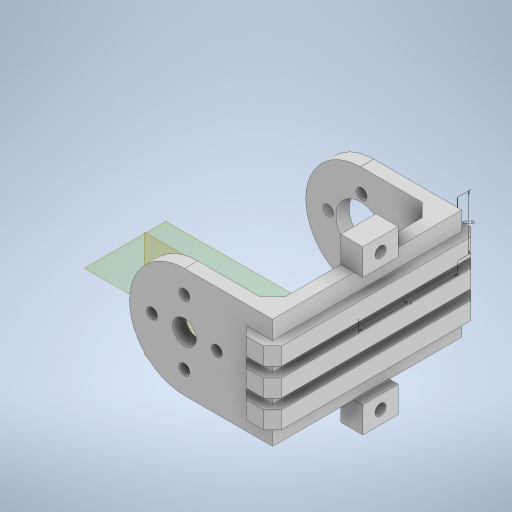
# Autodesk Inventor part: UnionCuerpo
Saved by Autodesk Inventor 2024 (Build 280153000, 153)
## iProperties
Created: 2024-03-17
Part Number: UnionCuerpo
Material: Genérico
Document SubType Name: Modeling
Designer: na_re
Density: 1 g/cm^3
Appearance: Valor por defecto
Author: na_re
Autodesk Inventor part; units mm, degrees
ref_plane "YZ Plane" through (0, 0, 0) normal (1, 0, 0) x (0, 1, 0)
ref_plane "XZ Plane" through (0, 0, 0) normal (0, 1, 0) x (-1, 0, 0)
ref_plane "XY Plane" through (0, 0, 0) normal (0, 0, 1) x (1, 0, 0)
ref_plane "Plano de trabajo1" through (0, 0, 0) normal (0, 0, 1) x (1, 0, 0)
sketch "Boceto1" plane through (0, 0, 0) normal (0, 0, 1) x (1, 0, 0)
  circle A0 centre (18.3423, 0) radius 1.2028 projected
  circle A1 centre (3.6423, 0) radius 1.2028 projected
  circle A2 centre (10.9923, -7.35) radius 1.2028 projected
  circle A3 centre (10.9923, 7.35) radius 1.2028 projected
  circle A4 centre (10.9923, 0) radius 10.9823 projected
  circle A5 centre (10.9923, 0) radius 2.7 projected
  circle A6 centre (10.9923, 0) radius 12.5
  line L0 (10.9923, 0) -> (22.9923, 0)
  line L1 (10.9923, 0) -> (10.9923, 12.5)
  line L2 (10.9923, 12.5) -> (22.9923, 12.5)
  line L3 (10.9923, 0) -> (10.9923, -12.5)
  line L4 (10.9923, -12.5) -> (22.9923, -12.5)
  line L5 (22.9923, -12.5) -> (22.9923, 12.5)
  point P0 (0, 0)
  dimension "d0" = 25
  dimension "d1" = 12
  dimension "d2" = 12
  constraints: 12 end point, 2 horizontal, 2 perpendicular, 2 point on circle, 2 vertical, 1 centre point, 1 coincident, 1 tangent
  measures "d0" diameter of A6
  measures "d1" distance of L0.start L0.end
  measures "d2" distance of L1.end L2.end
extrude "Extrusión1" add sketch "Boceto1" along normal blind 3 contours L0 A4 L3 A2 A5 A0 | A0 L0 A5 L1 A3 A4 | L0 L5 A6 L3 A4 | A4 L1 A6 L5 L0 | L1 A3 A5 L3 A2 A4 | A4 L3 A6 L1 | L2 L5 A6 | A6 L5 L4
sketch "Boceto2" plane through (22.9923, -12.5, 0) normal (1, 0, 0) x (0, 0, -1)
  line L0 (0, 0) -> (0, 25) projected
  line L1 (0, 25) -> (-3, 25) projected
  line L2 (-3, 0) -> (-3, 25) projected
  line L3 (0, 0) -> (-3, 0) projected
  point P0 (0, 12.5)
extrude "Extrusión2" add sketch "Boceto2" along normal blind 8
sketch "Boceto3" plane through (0, 0, 0) normal (0, 0, -1) x (-1, 0, 0)
  line L0 (-10.9923, -12.5) -> (-30.9923, -12.5) projected
  arc A0 (-10.9923, -12.5) -> (-10.9923, 12.5) centre (-10.9923, 0) ccw projected
  line L1 (-10.9923, 12.5) -> (-30.9923, 12.5) projected
  line L2 (-30.9923, -12.5) -> (-30.9923, 12.5) projected
  circle A1 centre (-10.9923, 0) radius 2.7 projected
  circle A2 centre (-10.9923, 7.35) radius 1.2028 projected
  circle A3 centre (-18.3423, 0) radius 1.2028 projected
  circle A4 centre (-3.6423, 0) radius 1.2028 projected
  circle A5 centre (-10.9923, -7.35) radius 1.2028 projected
  line L3 (-30.9923, 12.5) -> (-27.9923, 12.5)
  line L4 (-27.9923, 12.5) -> (-27.9923, -12.5)
  line L5 (-27.9923, -12.5) -> (-30.9923, -12.5)
  line L6 (-30.9923, -12.5) -> (-30.9923, 12.5)
  point P0 (0, 0)
  dimension "d7" = 3
  constraints: 8 end point, 2 parallel, 1 horizontal, 1 perpendicular, 1 point on line
  measures "d7" distance of L4.end L5.end
extrude "Extrusión3" add sketch "Boceto3" along normal blind 42 contours L0 L2 L1 L4
sketch "Boceto4" plane through (27.9923, -12.5, 0) normal (-1, 0, 0) x (0, 0, 1)
  line L0 (-42, 0) -> (-42, 25) projected
  line L1 (0, 25) -> (0, 0) projected
  line L2 (0, 25) -> (-42, 25) projected
  line L3 (-42, 0) -> (-42, 25) projected
  line L4 (0, 0) -> (-42, 0) projected
  line L5 (-42, 0) -> (-40, 0)
  line L6 (-40, 0) -> (-40, 25)
  line L7 (-40, 25) -> (-42, 25)
  line L8 (-42, 25) -> (-42, 0)
  point P0 (0, 12.5)
  dimension "d10" = 2
  constraints: 8 end point, 2 parallel, 1 horizontal, 1 perpendicular, 1 point on line
  measures "d10" distance of L7.end L6.end
extrude "Extrusión4" add sketch "Boceto4" along normal blind 30 contours L0 L2 L6 L4
sketch "Boceto5" plane through (0, 0, -42) normal (0, 0, -1) x (-1, 0, 0)
  line L0 (24.4501, 12.6367) -> (24.5578, -12.3277) projected
  line L1 (-11.0672, 12.4835) -> (24.4501, 12.6367) projected
  arc A0 (-11.0672, 12.4835) -> (-10.9596, -12.4809) centre (-11.0134, 0.0013) ccw projected
  line L2 (-10.9596, -12.4809) -> (24.5578, -12.3277) projected
  circle A1 centre (-3.6676, 0.2495) radius 1.2028 projected
  circle A2 centre (-11.0134, 0.0013) radius 2.7 projected
  circle A3 centre (-10.7652, -7.3445) radius 1.2028 projected
  circle A4 centre (-11.2616, 7.3471) radius 1.2028 projected
  circle A5 centre (-18.3592, -0.2469) radius 1.2028 projected
  line L3 (-30.9923, 12.5) -> (2.0077, 12.5) projected
  line L4 (-11.0672, 12.4835) -> (2.0077, 12.5)
  line L5 (2.0391, -12.4248) -> (2.0077, 12.5)
  line L6 (-10.9596, -12.4809) -> (2.0391, -12.4248)
  line L7 (-11.0672, 12.4835) -> (2.0077, 12.5)
  circle A6 centre (-11.0134, 0.0013) radius 12.4823
  line L8 (-10.7652, -7.3445) -> (-10.7652, -14.8497)
  line L9 (-10.7652, -14.8497) -> (6.2045, -14.8497)
  line L10 (6.2045, -14.8497) -> (6.2045, 15.7882)
  line L11 (6.2045, 15.7882) -> (-10.7652, 15.7882)
  line L12 (-10.7652, 15.7882) -> (-11.2616, 7.3471)
  point P0 (0, 0)
  point P1 (-7.2489, 12.5)
  point P2 (-10.991, 12.4836)
  point P3 (-10.9817, -12.481)
  point P4 (-10.9586, 12.5)
  point P5 (6.2045, 12.558)
  point P6 (6.2045, -12.4069)
  point P7 (-10.7652, -12.48)
  point P8 (-10.9595, 12.484)
  point P9 (-10.9595, 12.4837)
  point P10 (-10.9596, 12.4835)
  point P11 (-10.991, 12.4836)
  point P12 (-10.7652, -12.4785)
  point P13 (-11.0672, 12.4835)
  constraints: 18 end point, 4 perpendicular, 2 point on line, 1 coincident, 1 collinear, 1 vertical, 3 other
extrude "Extrusión5" cut sketch "Boceto5" against normal blind 25 contours L10 L2 L5 L3 L1 | L1 L3 L12 L11 L10 | L10 L9 L8 L2 | L3 L4 L1 | L1 L12 L3 | L2 A6 L4 L5 | A1 | A2 | A3 | A4 | A5
sketch "Boceto8" plane through (10.9923, -12.5, 0) normal (0, -1, 0) x (1, 0, 0)
  line L0 (-0.2271, -40) -> (-0.2271, -42) projected
  line L1 (20, -42) -> (-0.2271, -42) projected
  line L2 (20, 3) -> (20, -42) projected
  line L3 (0, 3) -> (20, 3) projected
  line L4 (0, 0) -> (0, 3) projected
  line L5 (0, 0) -> (17, 0) projected
  line L6 (17, 0) -> (17, -40) projected
  line L7 (17, -40) -> (-0.2271, -40) projected
  line L8 (20, -42) -> (20, -19.5)
  line L9 (20, 3) -> (20, -42) projected
  line L10 (20, -19.5) -> (20, -23.5)
  line L11 (20, -23.5) -> (20, -15.5)
  line L12 (20, -15.5) -> (17, -15.5)
  line L13 (20, -23.5) -> (17, -23.5)
  point P0 (-10.9923, 0)
  dimension "d29" = 22.5
  dimension "d30" = 4
  dimension "d31" = 8
  constraints: 10 end point, 4 point on line, 2 perpendicular, 1 midpoint
  measures "d29" distance of L1.start L8.end
  measures "d30" distance of L8.end L10.end
  measures "d31" distance of L10.end L11.end
extrude "Extrusión8" add sketch "Boceto8" along normal blind 6 contours L6 L12 L2 L13
ref_plane "Plano de trabajo2" through (-0.8313, -11.6464, -27.56) normal (0.0047593, -0.9999887, 0) x (0.9999887, 0.0047593, 0)
sketch "Boceto9" plane through (30.9923, -12.5, 0) normal (1, 0, 0) x (0, 0, -1)
  line L0 (-3, 25) -> (42, 25) projected
  line L1 (-3, 25) -> (-3, 0) projected
  line L2 (-3, 0) -> (15.5, 0) projected
  line L3 (15.5, 0) -> (15.5, -6) projected
  line L4 (23.5, -6) -> (15.5, -6) projected
  line L5 (23.5, 0) -> (23.5, -6) projected
  line L6 (23.5, 0) -> (42, 0) projected
  line L7 (42, 25) -> (42, 0) projected
  line L8 (23.5, 0) -> (23.5, 25)
  line L9 (23.5, 25) -> (23.5, 31)
  line L10 (23.5, 31) -> (15.5, 31)
  line L11 (15.5, 31) -> (15.5, 25)
  point P0 (0, 12.5)
  dimension "d34" = 6
  constraints: 8 end point, 3 perpendicular, 2 point on line, 1 vertical
  measures "d34" distance of L8.end L9.end
extrude "Extrusión9" add sketch "Boceto9" against normal blind 3 contours L11 L10 L9 L0
sketch "Boceto10" plane through (27.9923, -12.5, 0) normal (-1, 0, 0) x (0, 0, 1)
  line L0 (-40, 25) -> (-40, 0) projected
  line L1 (-23.5, 0) -> (-40, 0) projected
  line L2 (-23.5, 0) -> (-23.5, -6) projected
  line L3 (-15.5, -6) -> (-23.5, -6) projected
  line L4 (-15.5, 0) -> (-15.5, -6) projected
  line L5 (0, 0) -> (-15.5, 0) projected
  line L6 (0, 25) -> (0, 0) projected
  line L7 (0, 25) -> (-15.5, 25) projected
  line L8 (-15.5, 25) -> (-15.5, 31) projected
  line L9 (-15.5, 31) -> (-23.5, 31) projected
  line L10 (-23.5, 31) -> (-23.5, 25) projected
  line L11 (-23.5, 25) -> (-40, 25) projected
  line L12 (-15.5, -3) -> (-19.5, -3)
  line L13 (-19.5, -3) -> (-19.5, 28)
  circle A0 centre (-19.5, -3) radius 1.25
  circle A1 centre (-19.5, 28) radius 1.25
  point P0 (0, 12.5)
  dimension "d37" = 2.5
  dimension "d38" = 2.5
  constraints: 4 end point, 2 centre point, 2 coincident, 1 horizontal, 1 midpoint, 1 perpendicular
  measures "d37" diameter of A0
  measures "d38" diameter of A1
extrude "Extrusión10" cut sketch "Boceto10" against normal blind 3 contours A0 L13 L12 | L12 L13 A0 | A1
sketch "Boceto11" plane through (27.9923, -12.5, 0) normal (-1, 0, 0) x (0, 0, 1)
  line L0 (-42, 25) -> (-42, 0) projected
  line L1 (-42, 25) -> (-42, 12.5)
  line L2 (-42, 12.5) -> (-19.5, 12.5)
  line L3 (3, 13.7028) -> (3, 11.2972) projected
  line L4 (-19.5, 12.5) -> (-19.5, 25)
  point P0 (0, 12.5)
  dimension "d41" = 12.5
  dimension "d42" = 22.5
  constraints: 6 end point, 1 midpoint, 1 perpendicular, 1 vertical
  measures "d41" distance of L0.start L1.end
  measures "d42" distance of L1.end L2.end
sketch "Boceto12" plane through (27.9923, -12.5, -40) normal (0, 0, 1) x (1, 0, 0)
  circle A0 centre (-16.9789, 12.5013) radius 5.6 projected
  circle A1 centre (-16.9789, 12.5013) radius 5.6 projected
  circle A2 centre (-16.9789, 12.5013) radius 2.7 projected
  point P0 (-27.9923, 12.5)
extrude "Extrusión11" cut sketch "Boceto12" against normal blind 10
sketch "Boceto13" plane through (27.9923, -12.5, -40) normal (0, 0, 1) x (1, 0, 0)
  circle A0 centre (-16.9789, 12.5013) radius 5.6 projected
  line L0 (-17.0337, 25) -> (-17.0328, 24.9835) projected
  arc A1 (-17.0328, 24.9835) -> (-17.2271, 0.0215) centre (-16.9789, 12.5013) ccw projected
  line L1 (-17.2271, 0.0215) -> (-17.2271, 0) projected
  line L2 (0, 0) -> (-17.2271, 0) projected
  line L3 (0, 25) -> (0, 0) projected
  line L4 (0, 25) -> (-17.0337, 25) projected
  circle A2 centre (-9.6331, 12.2531) radius 1.2028 projected
  circle A3 centre (-16.7307, 19.8471) radius 1.2028 projected
  circle A4 centre (-17.2271, 5.1555) radius 1.2028 projected
  circle A5 centre (-24.3247, 12.7495) radius 1.2028 projected
  point P0 (-27.9923, 12.5)
extrude "Extrusión12" add sketch "Boceto13" along normal blind 6
sketch "Boceto15" plane through (27.9923, -12.5, -34) normal (0, 0, 1) x (1, 0, 0)
  line L0 (-17.0337, 25) -> (-17.0328, 24.9835) projected
  arc A0 (-17.0328, 24.9835) -> (-17.2271, 0.0215) centre (-16.9789, 12.5013) ccw projected
  line L1 (-17.2271, 0.0215) -> (-17.2271, 0) projected
  line L2 (-17.2271, 0) -> (0, 0) projected
  line L3 (0, 25) -> (0, 0) projected
  line L4 (0, 25) -> (-17.0337, 25) projected
  circle A1 centre (-9.6331, 12.2531) radius 1.2028 projected
  circle A2 centre (-24.3247, 12.7495) radius 1.2028 projected
  circle A3 centre (-17.2271, 5.1555) radius 1.2028 projected
  circle A4 centre (-16.7307, 19.8471) radius 1.2028 projected
  circle A5 centre (-16.9789, 12.5013) radius 5.6 projected
  point P0 (-27.9923, 12.5)
extrude "Extrusión14" cut sketch "Boceto15" against normal blind 3
sketch "Boceto16" plane through (0, 0, -42) normal (0, 0, -1) x (-1, 0, 0)
  circle A0 centre (-11.0134, 0.0013) radius 5.6 projected
  line L0 (-10.9596, 12.4835) -> (-10.9586, 12.5) projected
  line L1 (-30.9923, 12.5) -> (-10.9586, 12.5) projected
  line L2 (-30.9923, 12.5) -> (-30.9923, -12.5) projected
  line L3 (-30.9923, -12.5) -> (-10.7652, -12.5) projected
  line L4 (-10.7652, -12.5) -> (-10.7652, -12.4785) projected
  arc A1 (-10.7652, -12.4785) -> (-10.9596, 12.4835) centre (-11.0134, 0.0013) ccw projected
  circle A2 centre (-3.6676, 0.2495) radius 1.2028 projected
  circle A3 centre (-10.7652, -7.3445) radius 1.2028 projected
  circle A4 centre (-11.2616, 7.3471) radius 1.2028 projected
  circle A5 centre (-18.3592, -0.2469) radius 1.2028 projected
  point P0 (0, 0)
extrude "Extrusión15" cut sketch "Boceto16" against normal blind 2
sketch "Boceto17" plane through (27.9923, -12.5, 0) normal (-1, 0, 0) x (0, 0, 1)
  line L0 (-23.5, 0) -> (-37, 0) projected
  line L1 (-23.5, 0) -> (-23.5, -6) projected
  line L2 (-15.5, -6) -> (-23.5, -6) projected
  line L3 (-15.5, 0) -> (-15.5, -6) projected
  line L4 (0, 0) -> (-15.5, 0) projected
  line L5 (0, 25) -> (0, 0) projected
  line L6 (0, 25) -> (-15.5, 25) projected
  line L7 (-15.5, 25) -> (-15.5, 31) projected
  line L8 (-15.5, 31) -> (-23.5, 31) projected
  line L9 (-23.5, 31) -> (-23.5, 25) projected
  line L10 (-23.5, 25) -> (-37, 25) projected
  line L11 (-37, 25) -> (-37, 0) projected
  circle A0 centre (-19.5, -3) radius 1.25 projected
  circle A1 centre (-19.5, 28) radius 1.25 projected
  line L12 (0, 0) -> (-3, 0)
  line L13 (-3, 0) -> (-3, 25)
  line L14 (-3, 25) -> (0, 25)
  line L15 (0, 25) -> (0, 0)
  line L16 (-37, 25) -> (-34, 25)
  line L17 (-34, 25) -> (-34, 0)
  line L18 (-34, 0) -> (-37, 0)
  line L19 (-37, 0) -> (-37, 25)
  point P0 (0, 12.5)
  dimension "d53" = 3
  dimension "d54" = 3
  constraints: 16 end point, 4 parallel, 2 horizontal, 2 perpendicular, 2 point on line
  measures "d53" distance of L13.end L14.end
  measures "d54" distance of L17.end L18.end
extrude "Extrusión16" add sketch "Boceto17" along normal blind 3 contours L0 L11 L10 L17 | L13 L6 L5 L4
chamfer "Chaflán1" distance 3 angle 45 2 edges at (24.9923, 0, -3) (24.9923, 0, -34)
sketch "Boceto18" plane through (30.9923, -12.5, 0) normal (1, 0, 0) x (0, 0, -1)
  line L0 (40, 0) -> (40, 25) projected
  line L1 (23.5, 25) -> (40, 25) projected
  line L2 (23.5, 25) -> (23.5, 31) projected
  line L3 (23.5, 31) -> (15.5, 31) projected
  line L4 (15.5, 31) -> (15.5, 25) projected
  line L5 (-3, 25) -> (15.5, 25) projected
  line L6 (-3, 25) -> (-3, 0) projected
  line L7 (-3, 0) -> (15.5, 0) projected
  line L8 (15.5, 0) -> (15.5, -6) projected
  line L9 (23.5, -6) -> (15.5, -6) projected
  line L10 (23.5, 0) -> (23.5, -6) projected
  line L11 (23.5, 0) -> (40, 0) projected
  circle A0 centre (19.5, 28) radius 1.25 projected
  circle A1 centre (19.5, -3) radius 1.25 projected
  line L12 (40, 25) -> (40, 12.5)
  line L13 (40, 12.5) -> (40, 18.75)
  line L14 (40, 18.75) -> (31.75, 18.75)
  line L15 (40, 12.5) -> (31.75, 12.5)
  line L16 (40, 12.5) -> (40, 6.25)
  line L17 (40, 0) -> (40, 25) projected
  line L18 (40, 6.25) -> (31.75, 6.25)
  line L19 (40, 18.75) -> (31.75, 18.75)
  line L20 (31.75, 18.75) -> (31.75, 20.75)
  line L21 (31.75, 20.75) -> (40, 20.75)
  line L22 (40, 20.75) -> (40, 18.75)
  line L23 (31.75, 18.75) -> (40, 18.75)
  line L24 (40, 18.75) -> (40, 16.75)
  line L25 (40, 16.75) -> (31.75, 16.75)
  line L26 (31.75, 16.75) -> (31.75, 18.75)
  line L27 (15.5, 25) -> (23.5, 25)
  line L28 (23.5, 25) -> (23.5, 31)
  line L29 (23.5, 31) -> (15.5, 31)
  line L30 (15.5, 31) -> (15.5, 25)
  line L31 (15.5, 0) -> (23.5, 0)
  line L32 (23.5, 0) -> (23.5, -6)
  line L33 (23.5, -6) -> (15.5, -6)
  line L34 (15.5, -6) -> (15.5, 0)
  circle A2 centre (19.5, 28) radius 1.25 projected
  circle A3 centre (19.5, 28) radius 1.25
  circle A4 centre (19.5, -3) radius 1.25
  line L35 (31.75, 12.5) -> (31.75, 14.5)
  line L36 (31.75, 12.5) -> (31.75, 10.5)
  line L37 (31.75, 10.5) -> (40, 10.5)
  line L38 (31.75, 14.5) -> (40, 14.5)
  line L39 (31.75, 6.25) -> (31.75, 8.25)
  line L40 (31.75, 8.25) -> (40, 8.25)
  line L41 (31.75, 6.25) -> (31.75, 4.25)
  line L42 (31.75, 4.25) -> (40, 4.25)
  line L43 (40, 25) -> (18.5, 25)
  line L44 (18.5, 25) -> (18.5, 0)
  line L45 (5.25, 20.75) -> (-3, 20.75)
  line L46 (-3, 16.75) -> (5.25, 16.75)
  line L47 (5.25, 10.5) -> (-3, 10.5)
  line L48 (5.25, 14.5) -> (-3, 14.5)
  line L49 (5.25, 8.25) -> (-3, 8.25)
  line L50 (5.25, 4.25) -> (-3, 4.25)
  line L51 (5.25, 20.75) -> (5.25, 16.75)
  line L52 (5.25, 14.5) -> (5.25, 10.5)
  line L53 (5.25, 8.25) -> (5.25, 4.25)
  line L54 (-3, 20.75) -> (-3, 16.75)
  line L55 (-3, 14.5) -> (-3, 10.5)
  line L56 (-3, 8.25) -> (-3, 4.25)
  line L57 (31.75, 20.75) -> (5.25, 20.75)
  line L58 (31.75, 16.75) -> (5.25, 16.75)
  line L59 (5.25, 14.5) -> (31.75, 14.5)
  line L60 (31.75, 10.5) -> (5.25, 10.5)
  line L61 (5.25, 8.25) -> (31.75, 8.25)
  line L62 (31.75, 4.25) -> (5.25, 4.25)
  point P0 (0, 12.5)
  point P1 (40, 4.25)
  dimension "d60" = 12.5
  dimension "d61" = 6.25
  dimension "d62" = 8.25
  dimension "d63" = 6.25
  dimension "d64" = 2
  dimension "d65" = 2
  dimension "d66" = 2
  dimension "d67" = 2
  dimension "d68" = 2
  dimension "d69" = 2
  dimension "d70" = 21.5
  constraints: 100 end point, 12 perpendicular, 12 symmetric about line, 10 parallel, 7 collinear, 6 horizontal, 4 point on line, 3 vertical, 2 centre point, 2 coincident, 2 midpoint, 1 concentric, 7 other
  measures "d60" distance of L0.end L12.end
  measures "d61" distance of L12.end L13.end
  measures "d62" distance of L13.end L14.end
  measures "d63" distance of L12.end L16.end
  measures "d64" distance of L19.end L20.end
  measures "d65" distance of L23.end L24.end
  measures "d66" distance of L15.end L35.end
  measures "d67" distance of L15.end L36.end
  measures "d68" distance of L18.end L39.end
  measures "d69" distance of L18.end L41.end
  measures "d70" distance of L0.end L43.end
extrude "Extrusión17" add sketch "Boceto18" along normal blind 2 contours L42 L41 L18 L0 | L10 L9 L8 L31 | L18 L39 L40 L0 | L62 L44 L61 L39 L41 | L62 L53 L61 L44 | L37 L36 L15 L0 | L50 L6 L49 L53 | L15 L35 L38 L0 | L60 L44 L59 L35 L36 | L60 L52 L59 L44 | L47 L6 L48 L52 | L25 L26 L14 L0 | L58 L51 L57 L44 | L44 L57 L20 L26 L58 | L14 L20 L21 L0 | L46 L6 L45 L51 | L27 L4 L3 L2
sketch "Boceto19" plane through (0, 0, -40) normal (0, 0, -1) x (-1, 0, 0)
  line L0 (-30.9923, 8.25) -> (-32.9923, 8.25) projected
  line L1 (-32.9923, 8.25) -> (-24.9923, 8.25)
  line L2 (-24.9923, -12.5) -> (-24.9923, 12.5) projected
  line L3 (-30.9923, 4.25) -> (-32.9923, 4.25) projected
  line L4 (-30.9923, 4.25) -> (-24.9923, 4.25)
  line L5 (-24.9923, 4.25) -> (-24.9923, 8.25)
  line L6 (-32.9923, 4.25) -> (-32.9923, 8.25) projected
  line L7 (-32.9923, 4.25) -> (-32.9923, 8.25)
  line L8 (-32.9923, 4.25) -> (-30.9923, 4.25)
  line L9 (-32.9923, -2) -> (-32.9923, 2) projected
  line L10 (-32.9923, 2) -> (-24.9923, 2)
  line L11 (-24.9923, 2) -> (-24.9923, -2)
  line L12 (-24.9923, -2) -> (-32.9923, -2)
  line L13 (-32.9923, -2) -> (-32.9923, 2)
  line L14 (-30.9923, -4.25) -> (-32.9923, -4.25) projected
  line L15 (-32.9923, -4.25) -> (-24.9923, -4.25)
  line L16 (-24.9923, -4.25) -> (-24.9923, -8.25)
  line L17 (-24.9923, -8.25) -> (-32.9923, -8.25)
  line L18 (-32.9923, -8.25) -> (-32.9923, -4.25)
  point P0 (0, 0)
  dimension "d73" = 4
  constraints: 26 end point, 5 equal length, 5 horizontal, 3 perpendicular, 3 point on line
  measures "d73" distance of L15.end L16.end
extrude "Extrusión18" add sketch "Boceto19" along normal blind 2
sketch "Boceto20" plane through (0, 0, 3) normal (0, 0, 1) x (1, 0, 0)
  line L0 (32.9923, 8.25) -> (32.9923, 4.25) projected
  line L1 (24.9923, 4.25) -> (30.9923, 4.25) projected
  line L2 (32.9923, 8.25) -> (24.9923, 8.25)
  line L3 (24.9923, 8.25) -> (24.9923, 4.25)
  line L4 (24.9923, 4.25) -> (32.9923, 4.25)
  line L5 (32.9923, 4.25) -> (32.9923, 8.25)
  line L6 (32.9923, -2) -> (24.9923, -2) projected
  line L7 (32.9923, 2) -> (24.9923, 2)
  line L8 (24.9923, 2) -> (24.9923, -2)
  line L9 (24.9923, -2) -> (32.9923, -2)
  line L10 (32.9923, -2) -> (32.9923, 2)
  line L11 (30.9923, -4.25) -> (24.9923, -4.25) projected
  line L12 (32.9923, -8.2413) -> (24.9923, -8.2413)
  line L13 (24.9923, -8.2413) -> (24.9923, -4.25)
  line L14 (24.9923, -4.25) -> (32.9923, -4.25)
  line L15 (32.9923, -4.25) -> (32.9923, -8.2413)
  point P0 (0, 0)
  constraints: 24 end point, 6 parallel, 3 horizontal, 3 perpendicular, 1 point on line
extrude "Extrusión19" add sketch "Boceto20" along normal blind 2
chamfer "Chaflán2" distance 2 angle 45 6 edges at (32.9923, 6.25, -42) (32.9923, 0, -42) (32.9923, -6.25, -42) (32.9923, 6.25, 5) (32.9923, 0, 5) (32.9923, -6.2457, 5)
chamfer "Chaflán3" distance 2 angle 45 6 edges at (24.9923, 6.25, -42) (24.9923, 0, -42) (24.9923, -6.25, -42) (24.9923, 6.25, 5) (24.9923, 0, 5) (24.9923, -6.2457, 5)
